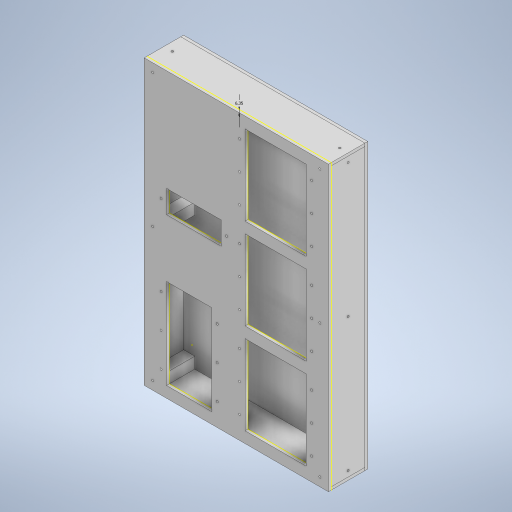
# Autodesk Inventor part: Faceplate
Saved by Autodesk Inventor 2024 (Build 280153020, 153B)
## iProperties
Created: 2023-08-04
Part Number: Faceplate
Material: Generic
Document SubType Name: Modeling
Designer: torban
Density: 1 g/cm^3
Appearance: Default
Author: torban
Autodesk Inventor part; units mm, degrees
ref_plane "YZ Plane" through (0, 0, 0) normal (1, 0, 0) x (0, 1, 0)
ref_plane "XZ Plane" through (0, 0, 0) normal (0, 1, 0) x (-1, 0, 0)
ref_plane "XY Plane" through (0, 0, 0) normal (0, 0, 1) x (1, 0, 0)
ref_plane "Work Plane1" through (0, 0, 0) normal (0, 0, 1) x (1, 0, 0)
sketch "Sketch1" plane through (0, 0, 0) normal (0, 0, 1) x (1, 0, 0)
  line L0 (181.4064, -95) -> (181.4064, -88.65)
  line L1 (181.4064, -88.65) -> (204.0936, -88.65)
  line L2 (204.0936, -88.65) -> (204.0936, -95)
  line L3 (204.0936, -95) -> (181.4064, -95)
  circle A0 centre (273, -11.325) radius 2.345
  circle A1 centre (112.5, -11.325) radius 2.345
  circle A2 centre (112.5, -75) radius 2.345
  circle A3 centre (273, -75) radius 2.345
  circle A4 centre (273, 52.35) radius 2.345
  circle A5 centre (112.5, 52.35) radius 2.345
  line L4 (187.75, -99) -> (197.75, -99)
  line L5 (197.75, -99) -> (197.75, -95)
  line L6 (197.75, -95) -> (204.0936, -95)
  line L7 (204.0936, -95) -> (204.0936, -88.65)
  spline S0 degree 2 poles (204.0936, -88.65) (209.94, -83.9409) (224.5027, -70.7595) knots 0 0 0 2.714255 2.714255 2.714255 weights 1 1.11961 1
  line L8 (224.5027, -70.7595) -> (255.1779, -70.7595)
  line L9 (255.1779, -70.7595) -> (255.1779, 72.35)
  line L10 (255.1779, 72.35) -> (260.5, 72.35)
  line L11 (260.5, 72.35) -> (285.5, 72.35)
  line L12 (285.5, 72.35) -> (285.5, -100)
  line L13 (285.5, -100) -> (260.5, -100)
  line L14 (260.5, -100) -> (125, -100)
  line L15 (125, -100) -> (125, 72.35)
  line L16 (100, 72.35) -> (125, 72.35)
  line L17 (100, -100) -> (100, 72.35)
  line L18 (125, -100) -> (100, -100)
  line L19 (187.75, -95) -> (187.75, -99)
  line L20 (181.4064, -95) -> (187.75, -95)
  line L21 (181.4064, -88.65) -> (181.4064, -95)
  spline S1 degree 2 poles (160.9973, -70.7595) (175.56, -83.9409) (181.4064, -88.65) knots 0 0 0 2.714255 2.714255 2.714255 weights 1 1.11961 1
  line L22 (130.3221, -70.7595) -> (160.9973, -70.7595)
  line L23 (130.3221, 72.35) -> (130.3221, -70.7595)
  line L24 (125, 72.35) -> (130.3221, 72.35)
  line L25 (260.5, 72.35) -> (260.5, -100)
  line L26 (260.5, 77.35) -> (260.5, 72.35)
  line L27 (285.5, 72.35) -> (260.5, 72.35)
  line L28 (285.5, 77.35) -> (285.5, 72.35)
  line L29 (260.5, 77.35) -> (285.5, 77.35)
  line L30 (125, 77.35) -> (260.5, 77.35)
  line L31 (125, 72.35) -> (125, 77.35)
  line L32 (125, 72.35) -> (100, 72.35)
  line L33 (100, 72.35) -> (100, 77.35)
  line L34 (100, 77.35) -> (125, 77.35)
  line L35 (260.5, 72.35) -> (125, 72.35)
  circle A6 centre (62.5, 75) radius 2.345
  circle A7 centre (-62.5, 75) radius 2.345
  circle A8 centre (-62.5, -75) radius 2.345
  circle A9 centre (62.5, -75) radius 2.345
  circle A10 centre (-62.5, 0) radius 2.345
  circle A11 centre (62.5, 0) radius 2.345
  circle A12 centre (-25, -60) radius 6
  circle A13 centre (0, -60) radius 6
  circle A14 centre (25, -60) radius 6
  circle A15 centre (0, 60) radius 8
  circle A16 centre (0, 20) radius 8
  circle A17 centre (0, -20) radius 8
  line L36 (-50, -100) -> (-50, 100)
  line L37 (-75, 100) -> (-50, 100)
  line L38 (-75, -100) -> (-75, 100)
  line L39 (-50, -100) -> (-75, -100)
  line L40 (50, -100) -> (-50, -100)
  line L41 (50, 100) -> (50, -100)
  line L42 (-50, 100) -> (50, 100)
  line L43 (75, -100) -> (50, -100)
  line L44 (75, 100) -> (75, -100)
  line L45 (50, 100) -> (75, 100)
  circle A18 centre (83.5, 254.7) radius 2.345
  circle A19 centre (-62.5, 254.7) radius 2.345
  line L46 (96, 229.7) -> (71, 229.7)
  line L47 (71, 229.7) -> (-50, 229.7)
  line L48 (-50, 229.7) -> (-75, 229.7)
  line L49 (-75, 229.7) -> (-75, 279.7)
  line L50 (-75, 279.7) -> (-50, 279.7)
  line L51 (-50, 279.7) -> (71, 279.7)
  line L52 (71, 279.7) -> (96, 279.7)
  line L53 (96, 279.7) -> (96, 229.7)
  line L54 (71, 279.7) -> (71, 229.7)
  line L55 (-50, 229.7) -> (-50, 279.7)
  line L56 (181.4064, 107.35) -> (181.4064, 113.7)
  line L57 (181.4064, 113.7) -> (204.0936, 113.7)
  line L58 (204.0936, 113.7) -> (204.0936, 107.35)
  line L59 (204.0936, 107.35) -> (181.4064, 107.35)
  circle A20 centre (273, 191.025) radius 2.345
  circle A21 centre (112.5, 191.025) radius 2.345
  circle A22 centre (112.5, 127.35) radius 2.345
  circle A23 centre (273, 127.35) radius 2.345
  circle A24 centre (273, 254.7) radius 2.345
  circle A25 centre (112.5, 254.7) radius 2.345
  line L60 (187.75, 103.35) -> (197.75, 103.35)
  line L61 (197.75, 103.35) -> (197.75, 107.35)
  line L62 (197.75, 107.35) -> (204.0936, 107.35)
  line L63 (204.0936, 107.35) -> (204.0936, 113.7)
  spline S2 degree 2 poles (204.0936, 113.7) (209.94, 118.4091) (224.5027, 131.5905) knots 0 0 0 2.714255 2.714255 2.714255 weights 1 1.11961 1
  line L64 (224.5027, 131.5905) -> (255.1779, 131.5905)
  line L65 (255.1779, 131.5905) -> (255.1779, 274.7)
  line L66 (255.1779, 274.7) -> (260.5, 274.7)
  line L67 (260.5, 274.7) -> (285.5, 274.7)
  line L68 (285.5, 274.7) -> (285.5, 102.35)
  line L69 (285.5, 102.35) -> (260.5, 102.35)
  line L70 (260.5, 102.35) -> (125, 102.35)
  line L71 (125, 102.35) -> (125, 274.7)
  line L72 (100, 274.7) -> (125, 274.7)
  line L73 (100, 102.35) -> (100, 274.7)
  line L74 (125, 102.35) -> (100, 102.35)
  line L75 (187.75, 107.35) -> (187.75, 103.35)
  line L76 (181.4064, 107.35) -> (187.75, 107.35)
  line L77 (181.4064, 113.7) -> (181.4064, 107.35)
  spline S3 degree 2 poles (160.9973, 131.5905) (175.56, 118.4091) (181.4064, 113.7) knots 0 0 0 2.714255 2.714255 2.714255 weights 1 1.11961 1
  line L78 (130.3221, 131.5905) -> (160.9973, 131.5905)
  line L79 (130.3221, 274.7) -> (130.3221, 131.5905)
  line L80 (125, 274.7) -> (130.3221, 274.7)
  line L81 (260.5, 274.7) -> (260.5, 102.35)
  line L82 (260.5, 279.7) -> (260.5, 274.7)
  line L83 (285.5, 274.7) -> (260.5, 274.7)
  line L84 (285.5, 279.7) -> (285.5, 274.7)
  line L85 (260.5, 279.7) -> (285.5, 279.7)
  line L86 (125, 279.7) -> (260.5, 279.7)
  line L87 (125, 274.7) -> (125, 279.7)
  line L88 (125, 274.7) -> (100, 274.7)
  line L89 (100, 274.7) -> (100, 279.7)
  line L90 (100, 279.7) -> (125, 279.7)
  line L91 (260.5, 274.7) -> (125, 274.7)
  line L92 (181.4064, 309.7) -> (181.4064, 316.05)
  line L93 (181.4064, 316.05) -> (204.0936, 316.05)
  line L94 (204.0936, 316.05) -> (204.0936, 309.7)
  line L95 (204.0936, 309.7) -> (181.4064, 309.7)
  circle A26 centre (273, 393.375) radius 2.345
  circle A27 centre (112.5, 393.375) radius 2.345
  circle A28 centre (112.5, 329.7) radius 2.345
  circle A29 centre (273, 329.7) radius 2.345
  circle A30 centre (273, 457.05) radius 2.345
  circle A31 centre (112.5, 457.05) radius 2.345
  line L96 (187.75, 305.7) -> (197.75, 305.7)
  line L97 (197.75, 305.7) -> (197.75, 309.7)
  line L98 (197.75, 309.7) -> (204.0936, 309.7)
  line L99 (204.0936, 309.7) -> (204.0936, 316.05)
  spline S4 degree 2 poles (204.0936, 316.05) (209.94, 320.7591) (224.5027, 333.9405) knots 0 0 0 2.714255 2.714255 2.714255 weights 1 1.11961 1
  line L100 (224.5027, 333.9405) -> (255.1779, 333.9405)
  line L101 (255.1779, 333.9405) -> (255.1779, 477.05)
  line L102 (255.1779, 477.05) -> (260.5, 477.05)
  line L103 (260.5, 477.05) -> (285.5, 477.05)
  line L104 (285.5, 477.05) -> (285.5, 304.7)
  line L105 (285.5, 304.7) -> (260.5, 304.7)
  line L106 (260.5, 304.7) -> (125, 304.7)
  line L107 (125, 304.7) -> (125, 477.05)
  line L108 (100, 477.05) -> (125, 477.05)
  line L109 (100, 304.7) -> (100, 477.05)
  line L110 (125, 304.7) -> (100, 304.7)
  line L111 (187.75, 309.7) -> (187.75, 305.7)
  line L112 (181.4064, 309.7) -> (187.75, 309.7)
  line L113 (181.4064, 316.05) -> (181.4064, 309.7)
  spline S5 degree 2 poles (160.9973, 333.9405) (175.56, 320.7591) (181.4064, 316.05) knots 0 0 0 2.714255 2.714255 2.714255 weights 1 1.11961 1
  line L114 (130.3221, 333.9405) -> (160.9973, 333.9405)
  line L115 (130.3221, 477.05) -> (130.3221, 333.9405)
  line L116 (125, 477.05) -> (130.3221, 477.05)
  line L117 (260.5, 477.05) -> (260.5, 304.7)
  line L118 (260.5, 482.05) -> (260.5, 477.05)
  line L119 (285.5, 477.05) -> (260.5, 477.05)
  line L120 (285.5, 482.05) -> (285.5, 477.05)
  line L121 (260.5, 482.05) -> (285.5, 482.05)
  line L122 (125, 482.05) -> (260.5, 482.05)
  line L123 (125, 477.05) -> (125, 482.05)
  line L124 (125, 477.05) -> (100, 477.05)
  line L125 (100, 477.05) -> (100, 482.05)
  line L126 (100, 482.05) -> (125, 482.05)
  line L127 (260.5, 477.05) -> (125, 477.05)
  line L128 (310.5, -125) -> (-100, -125)
  line L129 (-100, -125) -> (-100, 507.05)
  line L130 (-100, 507.05) -> (310.5, 507.05)
  line L131 (310.5, 507.05) -> (310.5, -125)
  point P0 (0, 0)
  point P1 (273, -100)
  point P2 (112.5, 482.05)
  dimension "d0" = 25
  dimension "d1" = 25
  dimension "d2" = 25
  dimension "d3" = 25
  constraints: 264 end point, 73 horizontal, 56 vertical, 32 centre point, 2 midpoint, 2 parallel, 1 perpendicular, 176 other
  measures "d0" distance from line of L128 point (273, -100)
  measures "d1" distance between parallel lines of L131 L12
  measures "d2" distance between parallel lines of L129 L38
  measures "d3" distance from line of L130 point (112.5, 482.05)
extrude "Extrusion1" add sketch "Sketch1" along normal blind 6.35 contours L15 L18 L17 L16 | L16 L33 L34 L31 | L26 L29 L28 L11 | L11 L12 L13 L25 | L39 L38 L37 L36 | L41 L45 L44 L43 | L46 L54 L52 L53 | L48 L49 L50 L55 | L71 L74 L73 L72 | L72 L89 L90 L87 | L82 L85 L84 L67 | L67 L68 L69 L81 | L107 L110 L109 L108 | L108 L125 L126 L123 | L118 L121 L120 L103 | L103 L104 L105 L117 | L128 L129 L130 L131
sketch "Sketch2" plane through (0, 0, 6.35) normal (0, 0, 1) x (1, 0, 0)
  circle A0 centre (273, 52.35) radius 2.345 projected
  circle A1 centre (273, -75) radius 2.345 projected
  circle A2 centre (273, -11.325) radius 2.345 projected
  line L0 (260.5, 77.35) -> (125, 77.35) projected
  line L1 (125, 77.35) -> (125, -100) projected
  line L2 (125, -100) -> (260.5, -100) projected
  line L3 (260.5, -100) -> (260.5, 77.35) projected
  circle A3 centre (112.5, 127.35) radius 2.345 projected
  circle A4 centre (112.5, 191.025) radius 2.345 projected
  circle A5 centre (112.5, 254.7) radius 2.345 projected
  circle A6 centre (273, 254.7) radius 2.345 projected
  circle A7 centre (273, 191.025) radius 2.345 projected
  circle A8 centre (273, 127.35) radius 2.345 projected
  circle A9 centre (112.5, 329.7) radius 2.345 projected
  circle A10 centre (112.5, 393.375) radius 2.345 projected
  circle A11 centre (112.5, 457.05) radius 2.345 projected
  circle A12 centre (273, 457.05) radius 2.345 projected
  circle A13 centre (273, 393.375) radius 2.345 projected
  circle A14 centre (273, 329.7) radius 2.345 projected
  circle A15 centre (62.5, 75) radius 2.345 projected
  circle A16 centre (62.5, -75) radius 2.345 projected
  circle A17 centre (62.5, 0) radius 2.345 projected
  circle A18 centre (-62.5, 0) radius 2.345 projected
  circle A19 centre (-62.5, -75) radius 2.345 projected
  circle A20 centre (-62.5, 75) radius 2.345 projected
  circle A21 centre (-62.5, 254.7) radius 2.345 projected
  circle A22 centre (83.5, 254.7) radius 2.345 projected
  line L4 (71, 229.7) -> (71, 279.7) projected
  line L5 (71, 279.7) -> (-50, 279.7) projected
  line L6 (-50, 279.7) -> (-50, 229.7) projected
  line L7 (-50, 229.7) -> (71, 229.7) projected
  line L8 (-50, 100) -> (-50, -100) projected
  line L9 (-50, -100) -> (50, -100) projected
  line L10 (50, -100) -> (50, 100) projected
  line L11 (50, 100) -> (-50, 100) projected
  line L12 (260.5, 304.7) -> (260.5, 482.05) projected
  line L13 (260.5, 482.05) -> (125, 482.05) projected
  line L14 (125, 482.05) -> (125, 304.7) projected
  line L15 (125, 304.7) -> (260.5, 304.7) projected
  line L16 (125, 279.7) -> (125, 102.35) projected
  line L17 (125, 102.35) -> (260.5, 102.35) projected
  line L18 (260.5, 102.35) -> (260.5, 279.7) projected
  line L19 (260.5, 279.7) -> (125, 279.7) projected
  circle A23 centre (112.5, -11.325) radius 2.345 projected
  circle A24 centre (112.5, -75) radius 2.345 projected
  circle A25 centre (112.5, 52.35) radius 2.345 projected
  line L20 (310.5, 507.05) -> (310.5, -125) projected
  line L21 (310.5, -125) -> (-100, -125) projected
  line L22 (-100, -125) -> (-100, 507.05) projected
  line L23 (-100, 507.05) -> (310.5, 507.05) projected
  line L24 (-50.25, 279.95) -> (71.25, 279.95)
  line L25 (71.25, 279.95) -> (71.25, 229.45)
  line L26 (71.25, 229.45) -> (-50.25, 229.45)
  line L27 (-50.25, 229.45) -> (-50.25, 279.95)
  line L28 (124.75, 279.95) -> (124.75, 102.1)
  line L29 (124.75, 102.1) -> (260.75, 102.1)
  line L30 (260.75, 102.1) -> (260.75, 279.95)
  line L31 (260.75, 279.95) -> (124.75, 279.95)
  line L32 (260.75, 304.45) -> (260.75, 482.3)
  line L33 (260.75, 482.3) -> (124.75, 482.3)
  line L34 (124.75, 482.3) -> (124.75, 304.45)
  line L35 (124.75, 304.45) -> (260.75, 304.45)
  line L36 (-50.25, 100.25) -> (-50.25, -100.25)
  line L37 (-50.25, -100.25) -> (50.25, -100.25)
  line L38 (50.25, -100.25) -> (50.25, 100.25)
  line L39 (50.25, 100.25) -> (-50.25, 100.25)
  line L40 (124.75, -100.25) -> (124.75, 77.6)
  line L41 (124.75, 77.6) -> (260.75, 77.6)
  line L42 (260.75, 77.6) -> (260.75, -100.25)
  line L43 (260.75, -100.25) -> (124.75, -100.25)
  point P0 (0, 0)
  dimension "d6" = 0.25
  dimension "d7" = 0.25
  dimension "d8" = 0.25
  dimension "d9" = 0.25
  dimension "d10" = 0.25
  constraints: 40 end point, 15 other
  measures "d6" distance between parallel lines of L5 L24
  measures "d7" distance between parallel lines of L19 L31
  measures "d8" distance between parallel lines of L15 L35
  measures "d9" distance between parallel lines of L11 L39
  measures "d10" distance between parallel lines of L1 L40
extrude "Extrusion2" cut sketch "Sketch2" against normal blind 6.35 contours L24 L25 L26 L27 | L31 L30 L29 L28 | L35 L34 L33 L32 | L39 L38 L37 L36 | L40 L41 L42 L43
sketch "Sketch3" plane through (0, 0, 0) normal (0, 0, -1) x (-1, 0, 0)
  line L0 (-71.25, 279.95) -> (-71.25, 229.45) projected
  line L1 (-71.25, 229.45) -> (50.25, 229.45) projected
  line L2 (50.25, 229.45) -> (50.25, 279.95) projected
  line L3 (50.25, 279.95) -> (-71.25, 279.95) projected
  line L4 (-50.25, 100.25) -> (-50.25, -100.25) projected
  line L5 (-50.25, -100.25) -> (50.25, -100.25) projected
  line L6 (50.25, -100.25) -> (50.25, 100.25) projected
  line L7 (50.25, 100.25) -> (-50.25, 100.25) projected
  line L8 (-260.75, 279.95) -> (-260.75, 102.1) projected
  line L9 (-260.75, 102.1) -> (-124.75, 102.1) projected
  line L10 (-124.75, 102.1) -> (-124.75, 279.95) projected
  line L11 (-124.75, 279.95) -> (-260.75, 279.95) projected
  line L12 (-124.75, 77.6) -> (-260.75, 77.6) projected
  line L13 (-260.75, 77.6) -> (-260.75, -100.25) projected
  line L14 (-260.75, -100.25) -> (-124.75, -100.25) projected
  line L15 (-124.75, -100.25) -> (-124.75, 77.6) projected
  line L16 (-124.75, 304.45) -> (-124.75, 482.3) projected
  line L17 (-124.75, 482.3) -> (-260.75, 482.3) projected
  line L18 (-260.75, 482.3) -> (-260.75, 304.45) projected
  line L19 (-260.75, 304.45) -> (-124.75, 304.45) projected
  circle A0 centre (-273, 52.35) radius 2.345 projected
  circle A1 centre (-273, -75) radius 2.345 projected
  circle A2 centre (-273, -11.325) radius 2.345 projected
  circle A3 centre (-112.5, 127.35) radius 2.345 projected
  circle A4 centre (-112.5, 191.025) radius 2.345 projected
  circle A5 centre (-112.5, 254.7) radius 2.345 projected
  circle A6 centre (-273, 254.7) radius 2.345 projected
  circle A7 centre (-273, 191.025) radius 2.345 projected
  circle A8 centre (-273, 127.35) radius 2.345 projected
  circle A9 centre (-112.5, 329.7) radius 2.345 projected
  circle A10 centre (-112.5, 393.375) radius 2.345 projected
  circle A11 centre (-112.5, 457.05) radius 2.345 projected
  circle A12 centre (-273, 457.05) radius 2.345 projected
  circle A13 centre (-273, 393.375) radius 2.345 projected
  circle A14 centre (-273, 329.7) radius 2.345 projected
  circle A15 centre (-62.5, 75) radius 2.345 projected
  circle A16 centre (-62.5, -75) radius 2.345 projected
  circle A17 centre (-62.5, 0) radius 2.345 projected
  circle A18 centre (62.5, 0) radius 2.345 projected
  circle A19 centre (62.5, -75) radius 2.345 projected
  circle A20 centre (62.5, 75) radius 2.345 projected
  circle A21 centre (62.5, 254.7) radius 2.345 projected
  circle A22 centre (-83.5, 254.7) radius 2.345 projected
  circle A23 centre (-112.5, -11.325) radius 2.345 projected
  circle A24 centre (-112.5, -75) radius 2.345 projected
  circle A25 centre (-112.5, 52.35) radius 2.345 projected
  line L20 (-310.5, -125) -> (-310.5, 507.05) projected
  line L21 (-310.5, 507.05) -> (100, 507.05) projected
  line L22 (100, 507.05) -> (100, -125) projected
  line L23 (100, -125) -> (-310.5, -125) projected
  line L24 (93.65, 500.7) -> (-304.15, 500.7)
  line L25 (-304.15, 500.7) -> (-304.15, -118.65)
  line L26 (-304.15, -118.65) -> (93.65, -118.65)
  line L27 (93.65, -118.65) -> (93.65, 500.7)
  line L28 (-304.15, 500.7) -> (-310.5, 500.7)
  line L29 (93.65, 500.7) -> (100, 500.7)
  line L30 (-304.15, -118.65) -> (-310.5, -118.65)
  line L31 (93.65, -118.65) -> (100, -118.65)
  point P0 (0, 0)
  dimension "d13" = 6.35
  constraints: 16 end point, 6 point on line, 2 perpendicular, 3 other
  measures "d13" distance between parallel lines of L21 L24
extrude "Extrusion3" add sketch "Sketch3" along normal blind 75 separate body contours L20 L30 L26 L31 L22 L23 | L20 L21 L22 L29 L24 L28
extrude "Extrusion4" add sketch "Sketch3" along normal blind 75 separate body contours L20 L28 L25 L30 | L31 L27 L29 L22
sketch "Sketch5" plane through (0, 0, 0) normal (0, 0, -1) x (-1, 0, 0)
  line L0 (-310.5, 500.7) -> (100, 500.7) projected
  line L1 (-304.1734, 500.7) -> (-279.1734, 500.7)
  line L2 (-279.1734, 500.7) -> (-279.1734, 475.7)
  line L3 (-279.1734, 475.7) -> (-304.1734, 475.7)
  line L4 (-304.1734, 475.7) -> (-304.1734, 500.7)
  line L5 (93.6127, 500.7) -> (68.6127, 500.7)
  line L6 (68.6127, 500.7) -> (68.6127, 475.7)
  line L7 (68.6127, 475.7) -> (93.6127, 475.7)
  line L8 (93.6127, 475.7) -> (93.6127, 500.7)
  line L9 (100, -118.65) -> (-310.5, -118.65) projected
  line L10 (93.6127, -118.65) -> (68.6127, -118.65)
  line L11 (68.6127, -118.65) -> (68.6127, -93.65)
  line L12 (68.6127, -93.65) -> (93.6127, -93.65)
  line L13 (93.6127, -93.65) -> (93.6127, -118.65)
  line L14 (-304.1734, -118.65) -> (-279.1734, -118.65)
  line L15 (-279.1734, -118.65) -> (-279.1734, -93.65)
  line L16 (-279.1734, -93.65) -> (-304.1734, -93.65)
  line L17 (-304.1734, -93.65) -> (-304.1734, -118.65)
  point P0 (0, 0)
  point P1 (68.6127, -118.65)
  point P2 (68.6127, 500.7)
  dimension "d20" = 25
  dimension "d21" = 25
  dimension "d22" = 25
  dimension "d23" = 25
  dimension "d24" = 25
  dimension "d25" = 25
  dimension "d26" = 25
  dimension "d27" = 25
  constraints: 32 end point, 8 parallel, 6 point on line, 4 horizontal, 4 perpendicular
  measures "d20" distance of L2.end L3.end
  measures "d21" distance of L1.end L2.end
  measures "d22" distance of L7.end L6.end
  measures "d23" distance of L6.end L5.end
  measures "d24" distance of L11.end L12.end
  measures "d25" distance of L10.end L11.end
  measures "d26" distance of L16.end L15.end
  measures "d27" distance of L15.end L14.end
extrude "Extrusion6" add sketch "Sketch5" along normal up to surface (75 mm away) separate body
sketch "Sketch6" plane through (0, 0, 0) normal (0, 0, -1) x (-1, 0, 0)
  line L0 (100, 507.05) -> (100, -125) projected
  line L1 (100, 191.025) -> (-310.5, 191.025)
  line L2 (-310.5, -125) -> (-310.5, 507.05) projected
  line L3 (100, 203.525) -> (-310.5, 203.525)
  line L4 (-303.7847, 203.525) -> (-278.7847, 203.525)
  line L5 (-278.7847, 203.525) -> (-278.7847, 178.525)
  line L6 (-278.7847, 178.525) -> (-303.7847, 178.525)
  line L7 (-303.7847, 178.525) -> (-303.7847, 203.525)
  line L8 (93.65, 500.7) -> (93.65, -118.65) projected
  line L9 (93.65, 203.525) -> (68.65, 203.525)
  line L10 (68.65, 203.525) -> (68.65, 178.525)
  line L11 (68.65, 178.525) -> (93.65, 178.525)
  line L12 (93.65, 178.525) -> (93.65, 203.525)
  point P0 (0, 0)
  point P1 (68.65, 203.525)
  point P2 (93.65, 178.525)
  dimension "d30" = 12.5
  dimension "d31" = 25
  dimension "d32" = 25
  dimension "d33" = 25
  dimension "d34" = 25
  constraints: 20 end point, 5 parallel, 3 point on line, 2 horizontal, 2 midpoint, 2 perpendicular
  measures "d30" distance between parallel lines of L1 L3
  measures "d31" distance of L5.end L6.end
  measures "d32" distance of L4.end L5.end
  measures "d33" distance of L11.end L10.end
  measures "d34" distance of L10.end L9.end
extrude "Extrusion7" add sketch "Sketch6" along normal up to surface (75 mm away) separate body contours L8 L1 L10 L3 | L8 L11 L10 L1 | L5 L1 L7 L3 | L5 L6 L7 L1
sketch "Sketch7" plane through (0, 0, 0) normal (0, 0, -1) x (-1, 0, 0)
  line L0 (-71.25, 279.95) -> (-71.25, 229.45) projected
  line L1 (-71.25, 229.45) -> (50.25, 229.45) projected
  line L2 (50.25, 229.45) -> (50.25, 279.95) projected
  line L3 (50.25, 279.95) -> (-71.25, 279.95) projected
  line L4 (-50.25, 100.25) -> (-50.25, -100.25) projected
  line L5 (-50.25, -100.25) -> (50.25, -100.25) projected
  line L6 (50.25, -100.25) -> (50.25, 100.25) projected
  line L7 (50.25, 100.25) -> (-50.25, 100.25) projected
  line L8 (-260.75, 279.95) -> (-260.75, 102.1) projected
  line L9 (-260.75, 102.1) -> (-124.75, 102.1) projected
  line L10 (-124.75, 102.1) -> (-124.75, 279.95) projected
  line L11 (-124.75, 279.95) -> (-260.75, 279.95) projected
  line L12 (-124.75, 77.6) -> (-260.75, 77.6) projected
  line L13 (-260.75, 77.6) -> (-260.75, -100.25) projected
  line L14 (-260.75, -100.25) -> (-124.75, -100.25) projected
  line L15 (-124.75, -100.25) -> (-124.75, 77.6) projected
  line L16 (-124.75, 304.45) -> (-124.75, 482.3) projected
  line L17 (-124.75, 482.3) -> (-260.75, 482.3) projected
  line L18 (-260.75, 482.3) -> (-260.75, 304.45) projected
  line L19 (-260.75, 304.45) -> (-124.75, 304.45) projected
  circle A0 centre (-273, 52.35) radius 2.345 projected
  circle A1 centre (-273, -75) radius 2.345 projected
  circle A2 centre (-273, -11.325) radius 2.345 projected
  circle A3 centre (-112.5, 127.35) radius 2.345 projected
  circle A4 centre (-112.5, 191.025) radius 2.345 projected
  circle A5 centre (-112.5, 254.7) radius 2.345 projected
  circle A6 centre (-273, 254.7) radius 2.345 projected
  circle A7 centre (-273, 191.025) radius 2.345 projected
  circle A8 centre (-273, 127.35) radius 2.345 projected
  circle A9 centre (-112.5, 329.7) radius 2.345 projected
  circle A10 centre (-112.5, 393.375) radius 2.345 projected
  circle A11 centre (-112.5, 457.05) radius 2.345 projected
  circle A12 centre (-273, 457.05) radius 2.345 projected
  circle A13 centre (-273, 393.375) radius 2.345 projected
  circle A14 centre (-273, 329.7) radius 2.345 projected
  circle A15 centre (-62.5, 75) radius 2.345 projected
  circle A16 centre (-62.5, -75) radius 2.345 projected
  circle A17 centre (-62.5, 0) radius 2.345 projected
  circle A18 centre (62.5, 0) radius 2.345 projected
  circle A19 centre (62.5, -75) radius 2.345 projected
  circle A20 centre (62.5, 75) radius 2.345 projected
  circle A21 centre (62.5, 254.7) radius 2.345 projected
  circle A22 centre (-83.5, 254.7) radius 2.345 projected
  circle A23 centre (-112.5, -11.325) radius 2.345 projected
  circle A24 centre (-112.5, -75) radius 2.345 projected
  circle A25 centre (-112.5, 52.35) radius 2.345 projected
  line L20 (-310.5, -125) -> (-310.5, 507.05) projected
  line L21 (-310.5, 507.05) -> (100, 507.05) projected
  line L22 (100, 507.05) -> (100, -125) projected
  line L23 (100, -125) -> (-310.5, -125) projected
  line L24 (100, -125) -> (-310.5, -125) projected
  line L25 (-310.5, -125) -> (-310.5, -118.65) projected
  line L26 (-310.5, -118.65) -> (100, -118.65) projected
  line L27 (100, -118.65) -> (100, -125) projected
  line L28 (-310.5, 507.05) -> (100, 507.05) projected
  line L29 (100, 507.05) -> (100, 500.7) projected
  line L30 (100, 500.7) -> (-310.5, 500.7) projected
  line L31 (-310.5, 500.7) -> (-310.5, 507.05) projected
  line L32 (-304.15, 500.7) -> (-304.15, -118.65) projected
  line L33 (-304.15, -118.65) -> (-310.5, -118.65) projected
  line L34 (-310.5, -118.65) -> (-310.5, 500.7) projected
  line L35 (-310.5, 500.7) -> (-304.15, 500.7) projected
  line L36 (93.65, -118.65) -> (93.65, 500.7) projected
  line L37 (93.65, 500.7) -> (100, 500.7) projected
  line L38 (100, 500.7) -> (100, -118.65) projected
  line L39 (100, -118.65) -> (93.65, -118.65) projected
  line L40 (93.6127, -118.65) -> (68.6127, -118.65) projected
  line L41 (68.6127, -118.65) -> (68.6127, -93.65) projected
  line L42 (68.6127, -93.65) -> (93.6127, -93.65) projected
  line L43 (93.6127, -93.65) -> (93.6127, -118.65) projected
  line L44 (-279.1734, 500.7) -> (-279.1734, 475.7) projected
  line L45 (-279.1734, 475.7) -> (-304.1734, 475.7) projected
  line L46 (-304.1734, 475.7) -> (-304.1734, 500.7) projected
  line L47 (-304.1734, 500.7) -> (-279.1734, 500.7) projected
  line L48 (-279.1734, -118.65) -> (-304.1734, -118.65) projected
  line L49 (-304.1734, -118.65) -> (-304.1734, -93.65) projected
  line L50 (-304.1734, -93.65) -> (-279.1734, -93.65) projected
  line L51 (-279.1734, -93.65) -> (-279.1734, -118.65) projected
  line L52 (93.6127, 500.7) -> (93.6127, 475.7) projected
  line L53 (93.6127, 475.7) -> (68.6127, 475.7) projected
  line L54 (68.6127, 475.7) -> (68.6127, 500.7) projected
  line L55 (68.6127, 500.7) -> (93.6127, 500.7) projected
  line L56 (-303.7847, 203.525) -> (-278.7847, 203.525) projected
  line L57 (-278.7847, 203.525) -> (-278.7847, 178.525) projected
  line L58 (-278.7847, 178.525) -> (-303.7847, 178.525) projected
  line L59 (-303.7847, 178.525) -> (-303.7847, 203.525) projected
  line L60 (93.65, 178.525) -> (68.65, 178.525) projected
  line L61 (68.65, 178.525) -> (68.65, 203.525) projected
  line L62 (68.65, 203.525) -> (93.65, 203.525) projected
  line L63 (93.65, 203.525) -> (93.65, 178.525) projected
  line L64 (-291.6734, 488.2) -> (81.1127, 488.2)
  line L65 (81.1127, 488.2) -> (81.1127, -106.15)
  line L66 (81.1127, -106.15) -> (-291.6734, -106.15)
  line L67 (-291.6734, -106.15) -> (-291.6734, 488.2)
  point P0 (0, 0)
  point P1 (81.1127, 191.025)
  point P2 (-291.6734, 191.025)
  dimension "d37" = 12.5
  dimension "d38" = 12.5
  dimension "d39" = 12.5
  dimension "d40" = 12.5
  constraints: 8 end point, 4 coincident, 2 midpoint, 2 parallel, 1 horizontal, 1 perpendicular
  measures "d37" distance between parallel lines of L66 L42
  measures "d38" distance between parallel lines of L41 L65
  measures "d39" distance between parallel lines of L44 L67
  measures "d40" distance between parallel lines of L45 L64
hole "Hole1" at (-81.1127, -106.15, 0) at (291.6734, -106.15, 0) at (291.6734, 191.025, 0) at (-81.1127, 191.025, 0) at (-81.1127, 488.2, 0) at (291.6734, 488.2, 0) direction (0, 0, 1) diameter 4.69 end through all bodies 1
sketch "Sketch8" plane through (-100, 500.7, 0) normal (0, -1, 0) x (1, 0, 0)
  line L0 (0, 0) -> (0, 6.35) projected
  line L1 (0, 6.35) -> (410.5, 6.35) projected
  line L2 (410.5, 6.35) -> (410.5, 0) projected
  line L3 (410.5, 0) -> (0, 0) projected
  line L4 (0, -75) -> (0, 0) projected
  line L5 (0, 0) -> (410.5, 0) projected
  line L6 (410.5, 0) -> (410.5, -75) projected
  line L7 (410.5, -75) -> (0, -75) projected
  line L8 (410.5, 0) -> (410.5, -75) projected
  line L9 (410.5, -75) -> (404.15, -75) projected
  line L10 (404.15, -75) -> (404.15, 0) projected
  line L11 (404.15, 0) -> (410.5, 0) projected
  line L12 (6.35, 0) -> (6.35, -75) projected
  line L13 (6.35, -75) -> (0, -75) projected
  line L14 (0, -75) -> (0, 0) projected
  line L15 (0, 0) -> (6.35, 0) projected
  line L16 (379.1734, 0) -> (404.1734, 0) projected
  line L17 (404.1734, 0) -> (404.1734, -75) projected
  line L18 (404.1734, -75) -> (379.1734, -75) projected
  line L19 (379.1734, -75) -> (379.1734, 0) projected
  line L20 (6.3873, 0) -> (31.3873, 0) projected
  line L21 (31.3873, 0) -> (31.3873, -75) projected
  line L22 (31.3873, -75) -> (6.3873, -75) projected
  line L23 (6.3873, -75) -> (6.3873, 0) projected
  line L24 (379.1734, -75) -> (404.1734, 0)
  line L25 (6.3873, -75) -> (31.3873, 0)
  point P0 (100, 0)
  point P1 (18.8873, -37.5)
  point P2 (391.6734, -37.5)
  constraints: 4 end point, 2 midpoint, 1 parallel, 1 other
hole "Hole2" at (291.6734, 500.7, -37.5) at (-81.1127, 500.7, -37.5) direction (0, 1, 0) diameter 4.69 end through all bodies 2
sketch "Sketch9" plane through (304.15, -118.65, 0) normal (-1, 0, 0) x (0, 0, 1)
  line L0 (0, 625.7) -> (6.35, 625.7) projected
  line L1 (6.35, 625.7) -> (6.35, -6.35) projected
  line L2 (6.35, -6.35) -> (0, -6.35) projected
  line L3 (0, -6.35) -> (0, 625.7) projected
  line L4 (0, 619.35) -> (-75, 619.35) projected
  line L5 (-75, 619.35) -> (-75, 625.7) projected
  line L6 (-75, 625.7) -> (0, 625.7) projected
  line L7 (0, 625.7) -> (0, 619.35) projected
  line L8 (-75, 0) -> (0, 0) projected
  line L9 (0, 0) -> (0, -6.35) projected
  line L10 (0, -6.35) -> (-75, -6.35) projected
  line L11 (-75, -6.35) -> (-75, 0) projected
  line L12 (0, 619.35) -> (0, 0) projected
  line L13 (0, 0) -> (-75, 0) projected
  line L14 (-75, 0) -> (-75, 619.35) projected
  line L15 (-75, 619.35) -> (0, 619.35) projected
  line L16 (0, 619.35) -> (0, 594.35) projected
  line L17 (0, 594.35) -> (-75, 594.35) projected
  line L18 (-75, 594.35) -> (-75, 619.35) projected
  line L19 (-75, 619.35) -> (0, 619.35) projected
  line L20 (-75, 25) -> (0, 25) projected
  line L21 (0, 25) -> (0, 0) projected
  line L22 (0, 0) -> (-75, 0) projected
  line L23 (-75, 0) -> (-75, 25) projected
  line L24 (0, 619.35) -> (-75, 619.35) projected
  line L25 (0, 594.35) -> (-75, 619.35)
  line L26 (0, 25) -> (-75, 0)
  line L27 (-75, 322.175) -> (-75, 297.175) projected
  line L28 (0, 297.175) -> (-75, 297.175) projected
  line L29 (0, 297.175) -> (0, 322.175) projected
  line L30 (0, 322.175) -> (-75, 322.175) projected
  line L31 (0, 322.175) -> (-75, 297.175)
  point P0 (0, 118.65)
  point P1 (-37.5, 309.675)
  point P2 (-37.5, 606.85)
  point P3 (-37.5, 12.5)
  constraints: 6 end point, 3 midpoint
hole "Hole3" at (304.15, -106.15, -37.5) at (304.15, 488.2, -37.5) at (304.15, 191.025, -37.5) direction (1, 0, 0) diameter 4.69 end through all bodies 3
sketch "Sketch4" plane through (0, 0, -75) normal (0, 0, -1) x (-1, 0, 0)
  line L0 (100, -125) -> (-310.5, -125) projected
  line L1 (-310.5, -125) -> (-310.5, -118.65) projected
  line L2 (-310.5, -118.65) -> (100, -118.65) projected
  line L3 (100, -118.65) -> (100, -125) projected
  line L4 (-310.5, 507.05) -> (100, 507.05) projected
  line L5 (100, 507.05) -> (100, 500.7) projected
  line L6 (100, 500.7) -> (-310.5, 500.7) projected
  line L7 (-310.5, 500.7) -> (-310.5, 507.05) projected
  line L8 (-304.15, 500.7) -> (-304.15, -118.65) projected
  line L9 (-304.15, -118.65) -> (-310.5, -118.65) projected
  line L10 (-310.5, -118.65) -> (-310.5, 500.7) projected
  line L11 (-310.5, 500.7) -> (-304.15, 500.7) projected
  line L12 (93.65, -118.65) -> (93.65, 500.7) projected
  line L13 (93.65, 500.7) -> (100, 500.7) projected
  line L14 (100, 500.7) -> (100, -118.65) projected
  line L15 (100, -118.65) -> (93.65, -118.65) projected
  line L16 (93.6127, -118.65) -> (68.6127, -118.65) projected
  line L17 (68.6127, -118.65) -> (68.6127, -93.65) projected
  line L18 (68.6127, -93.65) -> (93.6127, -93.65) projected
  line L19 (93.6127, -93.65) -> (93.6127, -118.65) projected
  line L20 (-279.1734, 475.7) -> (-304.1734, 475.7) projected
  line L21 (-304.1734, 475.7) -> (-304.1734, 500.7) projected
  line L22 (-304.1734, 500.7) -> (-279.1734, 500.7) projected
  line L23 (-279.1734, 500.7) -> (-279.1734, 475.7) projected
  line L24 (-279.1734, -118.65) -> (-304.1734, -118.65) projected
  line L25 (-304.1734, -118.65) -> (-304.1734, -93.65) projected
  line L26 (-304.1734, -93.65) -> (-279.1734, -93.65) projected
  line L27 (-279.1734, -93.65) -> (-279.1734, -118.65) projected
  line L28 (93.6127, 475.7) -> (68.6127, 475.7) projected
  line L29 (68.6127, 475.7) -> (68.6127, 500.7) projected
  line L30 (68.6127, 500.7) -> (93.6127, 500.7) projected
  line L31 (93.6127, 500.7) -> (93.6127, 475.7) projected
  line L32 (-303.7847, 203.525) -> (-278.7847, 203.525) projected
  line L33 (-278.7847, 203.525) -> (-278.7847, 178.525) projected
  line L34 (-278.7847, 178.525) -> (-303.7847, 178.525) projected
  line L35 (-303.7847, 178.525) -> (-303.7847, 203.525) projected
  line L36 (68.65, 178.525) -> (68.65, 203.525) projected
  line L37 (68.65, 203.525) -> (93.65, 203.525) projected
  line L38 (93.65, 203.525) -> (93.65, 178.525) projected
  line L39 (93.65, 178.525) -> (68.65, 178.525) projected
  point P0 (0, 0)
extrude "Extrusion5" add sketch "Sketch4" along normal blind 6.35 separate body contours L0 L1 L2 L3 | L2 L12 L6 L14 | L10 L6 L21 L20 L8 L26 L25 L2 | L2 L19 L18 L17 L27 L26 L8 L20 L23 L6 L29 L28 L31 L12 L37 L36 L39 | L6 L7 L4 L5 | L25 L26 L8 L2 | L2 L17 L18 L19 | L39 L36 L37 L12 | L8 L26 L27 L2 | L6 L8 L20 L21 | L31 L28 L29 L6 | L6 L23 L20 L8 | L32 L33 L34 L35
sketch "Sketch10" plane through (0, 0, -75) normal (0, 0, 1) x (1, 0, 0)
  line L0 (-100, 507.05) -> (310.5, 507.05) projected
  line L1 (310.5, 507.05) -> (310.5, 500.7) projected
  line L2 (310.5, 500.7) -> (-100, 500.7) projected
  line L3 (-100, 500.7) -> (-100, 507.05) projected
  line L4 (310.5, -125) -> (-100, -125) projected
  line L5 (-100, -125) -> (-100, -118.65) projected
  line L6 (-100, -118.65) -> (310.5, -118.65) projected
  line L7 (310.5, -118.65) -> (310.5, -125) projected
  line L8 (-93.65, 500.7) -> (-93.65, -118.65) projected
  line L9 (-93.65, -118.65) -> (-100, -118.65) projected
  line L10 (-100, -118.65) -> (-100, 500.7) projected
  line L11 (-100, 500.7) -> (-93.65, 500.7) projected
  line L12 (304.15, -118.65) -> (304.15, 500.7) projected
  line L13 (304.15, 500.7) -> (310.5, 500.7) projected
  line L14 (310.5, 500.7) -> (310.5, -118.65) projected
  line L15 (310.5, -118.65) -> (304.15, -118.65) projected
  line L16 (310.5, 507.05) -> (310.5, -125) projected
  line L17 (310.5, -125) -> (-100, -125) projected
  line L18 (-100, -125) -> (-100, 507.05) projected
  line L19 (-100, 507.05) -> (310.5, 507.05) projected
  line L20 (-68.6127, -118.65) -> (-93.6127, -118.65) projected
  line L21 (-93.6127, -118.65) -> (-93.6127, -93.65) projected
  line L22 (-93.6127, -93.65) -> (-68.6127, -93.65) projected
  line L23 (-68.6127, -93.65) -> (-68.6127, -118.65) projected
  line L24 (304.1734, 475.7) -> (279.1734, 475.7) projected
  line L25 (279.1734, 475.7) -> (279.1734, 500.7) projected
  line L26 (279.1734, 500.7) -> (304.1734, 500.7) projected
  line L27 (304.1734, 500.7) -> (304.1734, 475.7) projected
  line L28 (304.1734, -118.65) -> (279.1734, -118.65) projected
  line L29 (279.1734, -118.65) -> (279.1734, -93.65) projected
  line L30 (279.1734, -93.65) -> (304.1734, -93.65) projected
  line L31 (304.1734, -93.65) -> (304.1734, -118.65) projected
  line L32 (-68.6127, 475.7) -> (-93.6127, 475.7) projected
  line L33 (-93.6127, 475.7) -> (-93.6127, 500.7) projected
  line L34 (-93.6127, 500.7) -> (-68.6127, 500.7) projected
  line L35 (-68.6127, 500.7) -> (-68.6127, 475.7) projected
  line L36 (278.7847, 203.525) -> (303.7847, 203.525) projected
  line L37 (303.7847, 203.525) -> (303.7847, 178.525) projected
  line L38 (303.7847, 178.525) -> (278.7847, 178.525) projected
  line L39 (278.7847, 178.525) -> (278.7847, 203.525) projected
  line L40 (-68.65, 203.525) -> (-68.65, 178.525) projected
  line L41 (-68.65, 178.525) -> (-93.65, 178.525) projected
  line L42 (-93.65, 178.525) -> (-93.65, 203.525) projected
  line L43 (-93.65, 203.525) -> (-68.65, 203.525) projected
  line L44 (-93.6127, 488.2) -> (304.1734, 488.2)
  line L45 (291.6734, 500.7) -> (291.6734, -118.65)
  line L46 (304.1734, -106.15) -> (-93.6127, -106.15)
  line L47 (-81.1127, -118.65) -> (-81.1127, 500.7)
  point P0 (0, 0)
  point P1 (-81.1127, 488.2)
  point P2 (291.6734, 488.2)
  point P3 (291.6734, 191.025)
  point P4 (291.6734, -106.15)
  point P5 (-81.1127, -106.15)
  point P6 (-81.1127, 191.025)
  constraints: 10 midpoint, 8 end point, 8 point on line
hole "Hole4" at (-81.1127, 191.025, -75) at (-81.1127, -106.15, -75) at (291.6734, -106.15, -75) at (291.6734, 191.025, -75) at (291.6734, 488.2, -75) at (-81.1127, 488.2, -75) direction (0, 0, -1) diameter 4.69 end through all bodies 6
sketch "Sketch11" plane through (0, 0, 0) normal (0, 0, 1) x (1, 0, 0)
  circle A0 centre (291.6734, 488.2) radius 2.345 projected
  circle A1 centre (-81.1127, 488.2) radius 2.345 projected
  circle A2 centre (-81.1127, 191.025) radius 2.345 projected
  circle A3 centre (291.6734, 191.025) radius 2.345 projected
  circle A4 centre (291.6734, -106.15) radius 2.345 projected
  circle A5 centre (-81.1127, -106.15) radius 2.345 projected
  line L0 (71.25, 229.45) -> (71.25, 279.95) projected
  line L1 (71.25, 279.95) -> (-50.25, 279.95) projected
  line L2 (-50.25, 279.95) -> (-50.25, 229.45) projected
  line L3 (-50.25, 229.45) -> (71.25, 229.45) projected
  line L4 (50.25, -100.25) -> (50.25, 100.25) projected
  line L5 (50.25, 100.25) -> (-50.25, 100.25) projected
  line L6 (-50.25, 100.25) -> (-50.25, -100.25) projected
  line L7 (-50.25, -100.25) -> (50.25, -100.25) projected
  line L8 (260.75, 102.1) -> (260.75, 279.95) projected
  line L9 (260.75, 279.95) -> (124.75, 279.95) projected
  line L10 (124.75, 279.95) -> (124.75, 102.1) projected
  line L11 (124.75, 102.1) -> (260.75, 102.1) projected
  line L12 (260.75, 77.6) -> (124.75, 77.6) projected
  line L13 (124.75, 77.6) -> (124.75, -100.25) projected
  line L14 (124.75, -100.25) -> (260.75, -100.25) projected
  line L15 (260.75, -100.25) -> (260.75, 77.6) projected
  line L16 (124.75, 482.3) -> (124.75, 304.45) projected
  line L17 (124.75, 304.45) -> (260.75, 304.45) projected
  line L18 (260.75, 304.45) -> (260.75, 482.3) projected
  line L19 (260.75, 482.3) -> (124.75, 482.3) projected
  circle A6 centre (273, 52.35) radius 2.345 projected
  circle A7 centre (273, -75) radius 2.345 projected
  circle A8 centre (273, -11.325) radius 2.345 projected
  circle A9 centre (112.5, 127.35) radius 2.345 projected
  circle A10 centre (112.5, 191.025) radius 2.345 projected
  circle A11 centre (112.5, 254.7) radius 2.345 projected
  circle A12 centre (273, 254.7) radius 2.345 projected
  circle A13 centre (273, 191.025) radius 2.345 projected
  circle A14 centre (273, 127.35) radius 2.345 projected
  circle A15 centre (112.5, 329.7) radius 2.345 projected
  circle A16 centre (112.5, 393.375) radius 2.345 projected
  circle A17 centre (112.5, 457.05) radius 2.345 projected
  circle A18 centre (273, 457.05) radius 2.345 projected
  circle A19 centre (273, 393.375) radius 2.345 projected
  circle A20 centre (273, 329.7) radius 2.345 projected
  circle A21 centre (62.5, 75) radius 2.345 projected
  circle A22 centre (62.5, -75) radius 2.345 projected
  circle A23 centre (62.5, 0) radius 2.345 projected
  circle A24 centre (-62.5, 0) radius 2.345 projected
  circle A25 centre (-62.5, -75) radius 2.345 projected
  circle A26 centre (-62.5, 75) radius 2.345 projected
  circle A27 centre (-62.5, 254.7) radius 2.345 projected
  circle A28 centre (83.5, 254.7) radius 2.345 projected
  circle A29 centre (112.5, -11.325) radius 2.345 projected
  circle A30 centre (112.5, -75) radius 2.345 projected
  circle A31 centre (112.5, 52.35) radius 2.345 projected
  line L20 (310.5, 507.05) -> (310.5, -125) projected
  line L21 (310.5, -125) -> (-100, -125) projected
  line L22 (-100, -125) -> (-100, 507.05) projected
  line L23 (-100, 507.05) -> (310.5, 507.05) projected
  line L24 (-100, 507.05) -> (310.5, 507.05) projected
  line L25 (310.5, 507.05) -> (310.5, 500.7) projected
  line L26 (310.5, 500.7) -> (-100, 500.7) projected
  line L27 (-100, 500.7) -> (-100, 507.05) projected
  line L28 (310.5, -125) -> (-100, -125) projected
  line L29 (-100, -125) -> (-100, -118.65) projected
  line L30 (-100, -118.65) -> (310.5, -118.65) projected
  line L31 (310.5, -118.65) -> (310.5, -125) projected
  line L32 (-93.65, 500.7) -> (-93.65, -118.65) projected
  line L33 (-93.65, -118.65) -> (-100, -118.65) projected
  line L34 (-100, -118.65) -> (-100, 500.7) projected
  line L35 (-100, 500.7) -> (-93.65, 500.7) projected
  line L36 (304.15, -118.65) -> (304.15, 500.7) projected
  line L37 (304.15, 500.7) -> (310.5, 500.7) projected
  line L38 (310.5, 500.7) -> (310.5, -118.65) projected
  line L39 (310.5, -118.65) -> (304.15, -118.65) projected
  line L40 (-68.6127, -118.65) -> (-93.6127, -118.65) projected
  line L41 (-93.6127, -118.65) -> (-93.6127, -93.65) projected
  line L42 (-93.6127, -93.65) -> (-68.6127, -93.65) projected
  line L43 (-68.6127, -93.65) -> (-68.6127, -118.65) projected
  line L44 (279.1734, 475.7) -> (279.1734, 500.7) projected
  line L45 (279.1734, 500.7) -> (304.1734, 500.7) projected
  line L46 (304.1734, 500.7) -> (304.1734, 475.7) projected
  line L47 (304.1734, 475.7) -> (279.1734, 475.7) projected
  line L48 (304.1734, -118.65) -> (279.1734, -118.65) projected
  line L49 (279.1734, -118.65) -> (279.1734, -93.65) projected
  line L50 (279.1734, -93.65) -> (304.1734, -93.65) projected
  line L51 (304.1734, -93.65) -> (304.1734, -118.65) projected
  line L52 (-93.6127, 475.7) -> (-93.6127, 500.7) projected
  line L53 (-93.6127, 500.7) -> (-68.6127, 500.7) projected
  line L54 (-68.6127, 500.7) -> (-68.6127, 475.7) projected
  line L55 (-68.6127, 475.7) -> (-93.6127, 475.7) projected
  line L56 (278.7847, 203.525) -> (303.7847, 203.525) projected
  line L57 (303.7847, 203.525) -> (303.7847, 178.525) projected
  line L58 (303.7847, 178.525) -> (278.7847, 178.525) projected
  line L59 (278.7847, 178.525) -> (278.7847, 203.525) projected
  line L60 (-68.65, 178.525) -> (-93.65, 178.525) projected
  line L61 (-93.65, 178.525) -> (-93.65, 203.525) projected
  line L62 (-93.65, 203.525) -> (-68.65, 203.525) projected
  line L63 (-68.65, 203.525) -> (-68.65, 178.525) projected
  point P0 (0, 0)
extrude "Extrusion8" cut sketch "Sketch11" against normal through all contours A0 bodies 4
sketch "Sketch12" plane through (279.1734, 500.7, 0) normal (0, 1, 0) x (1, 0, 0)
  line L0 (-379.1734, -6.35) -> (-379.1734, 0) projected
  line L1 (-379.1734, 0) -> (31.3266, 0) projected
  line L2 (31.3266, 0) -> (31.3266, -6.35) projected
  line L3 (31.3266, -6.35) -> (-379.1734, -6.35) projected
  circle A0 centre (-360.286, 37.5) radius 2.345 projected
  circle A1 centre (12.5, 37.5) radius 2.345 projected
  line L4 (-379.1734, 0) -> (-379.1734, 75) projected
  line L5 (-379.1734, 75) -> (31.3266, 75) projected
  line L6 (31.3266, 75) -> (31.3266, 0) projected
  line L7 (31.3266, 0) -> (-379.1734, 0) projected
  line L8 (-372.8234, 75) -> (-372.8234, 0) projected
  line L9 (-372.8234, 0) -> (-379.1734, 0) projected
  line L10 (-379.1734, 0) -> (-379.1734, 75) projected
  line L11 (-379.1734, 75) -> (-372.8234, 75) projected
  line L12 (31.3266, 75) -> (31.3266, 0) projected
  line L13 (31.3266, 0) -> (24.9766, 0) projected
  line L14 (24.9766, 0) -> (24.9766, 75) projected
  line L15 (24.9766, 75) -> (31.3266, 75) projected
  line L16 (-379.1734, 75) -> (-379.1734, 81.35) projected
  line L17 (-379.1734, 81.35) -> (31.3266, 81.35) projected
  line L18 (31.3266, 81.35) -> (31.3266, 75) projected
  line L19 (31.3266, 75) -> (-379.1734, 75) projected
  line L20 (-347.786, 0) -> (-372.786, 0) projected
  line L21 (-372.786, 0) -> (-372.786, 75) projected
  line L22 (-372.786, 75) -> (-347.786, 75) projected
  line L23 (-347.786, 75) -> (-347.786, 0) projected
  line L24 (25, 0) -> (0, 0) projected
  line L25 (0, 0) -> (0, 75) projected
  line L26 (0, 75) -> (25, 75) projected
  line L27 (25, 75) -> (25, 0) projected
  point P0 (-279.1734, 0)
  constraints: 1 other
extrude "Extrusion9" cut sketch "Sketch12" against normal through all contours A1 bodies 4
sketch "Sketch13" plane through (304.1734, 475.7, 0) normal (1, 0, 0) x (0, 0, -1)
  line L0 (-6.35, 31.35) -> (0, 31.35) projected
  line L1 (0, 31.35) -> (0, -600.7) projected
  line L2 (0, -600.7) -> (-6.35, -600.7) projected
  line L3 (-6.35, -600.7) -> (-6.35, 31.35) projected
  line L4 (75, 25) -> (0, 25) projected
  line L5 (0, 25) -> (0, 31.35) projected
  line L6 (0, 31.35) -> (75, 31.35) projected
  line L7 (75, 31.35) -> (75, 25) projected
  line L8 (0, -594.35) -> (75, -594.35) projected
  line L9 (75, -594.35) -> (75, -600.7) projected
  line L10 (75, -600.7) -> (0, -600.7) projected
  line L11 (0, -600.7) -> (0, -594.35) projected
  circle A0 centre (37.5, -284.675) radius 2.345 projected
  circle A1 centre (37.5, 12.5) radius 2.345 projected
  circle A2 centre (37.5, -581.85) radius 2.345 projected
  line L12 (0, 25) -> (75, 25) projected
  line L13 (75, 25) -> (75, -594.35) projected
  line L14 (75, -594.35) -> (0, -594.35) projected
  line L15 (0, -594.35) -> (0, 25) projected
  line L16 (81.35, -600.7) -> (75, -600.7) projected
  line L17 (75, -600.7) -> (75, 31.35) projected
  line L18 (75, 31.35) -> (81.35, 31.35) projected
  line L19 (81.35, 31.35) -> (81.35, -600.7) projected
  line L20 (0, 0) -> (0, 25) projected
  line L21 (0, 25) -> (75, 25) projected
  line L22 (75, 25) -> (75, 0) projected
  line L23 (75, 0) -> (0, 0) projected
  line L24 (0, -594.35) -> (0, -569.35) projected
  line L25 (0, -569.35) -> (75, -569.35) projected
  line L26 (75, -569.35) -> (75, -594.35) projected
  line L27 (75, -594.35) -> (0, -594.35) projected
  point P0 (0, -475.7)
extrude "Extrusion10" cut sketch "Sketch13" against normal through all contours A1 bodies 4
body "Solid1"
body "Solid6"
